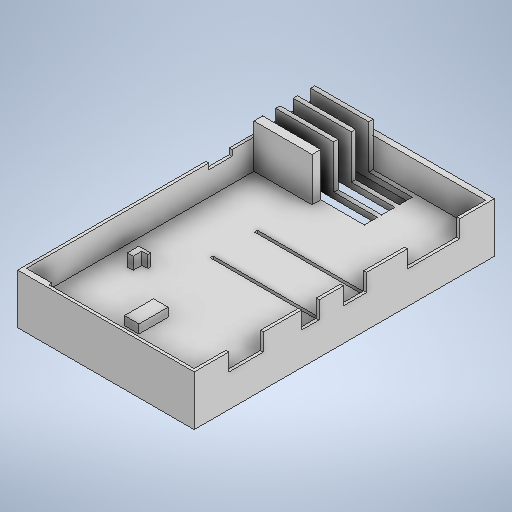
# Autodesk Inventor part: middle plate
Saved by Autodesk Inventor 2025.2 (Build 292293000, 293)
## iProperties
Created: 2025-04-04
Part Number: middle plate
Material: Generic
Document SubType Name: Modeling
Designer: joaki
Density: 1 g/cm^3
Appearance: Default
Author: joaki
Autodesk Inventor part; units mm, degrees
ref_plane "YZ Plane" through (0, 0, 0) normal (1, 0, 0) x (0, 1, 0)
ref_plane "XZ Plane" through (0, 0, 0) normal (0, 1, 0) x (-1, 0, 0)
ref_plane "XY Plane" through (0, 0, 0) normal (0, 0, 1) x (1, 0, 0)
sketch "Sketch1" plane through (0, 0, 0) normal (0, 1, 0) x (-1, 0, 0)
  line L0 (52.472, 79.0905) -> (-20.2681, 79.0905)
  line L1 (-20.2681, 79.0905) -> (-20.2681, -75.7549)
  line L2 (-20.2681, -75.7549) -> (52.472, -75.7549)
  line L3 (52.472, -75.7549) -> (52.472, 79.0905)
  line L4 (21.2319, -3.7723) -> (-15.2681, -3.7723)
  line L5 (-15.2681, -3.7723) -> (-15.2681, -4.7723)
  line L6 (-15.2681, -4.7723) -> (21.2319, -4.7723)
  line L7 (21.2319, -4.7723) -> (21.2319, -3.7723)
  line L8 (21.2319, -19.0703) -> (-15.2681, -19.0703)
  line L9 (-15.2681, -19.0703) -> (-15.2681, -20.0703)
  line L10 (-15.2681, -20.0703) -> (21.2319, -20.0703)
  line L11 (21.2319, -20.0703) -> (21.2319, -19.0703)
  point P0 (0, 0)
  point P1 (-15.2681, -4.2723)
  dimension "d0" = 36.5
  dimension "d1" = 1
  dimension "d2" = 1
  dimension "d3" = 36.5
  dimension "d4" = 14.298
  dimension "d7" = 5
  constraints: 24 end point, 6 parallel, 3 horizontal, 3 perpendicular, 1 midpoint
  measures "d0" distance of L5.end L6.end
  measures "d1" distance of L6.end L4.start
  measures "d2" distance of L10.end L8.start
  measures "d3" distance of L9.end L10.end
  measures "d4" distance between parallel lines of L6 L8
  measures "d7" distance from line of point (-15.268, -4.272) L1
extrude "Extrusion1" add sketch "Sketch1" along normal blind 2
sketch "Sketch3" plane through (0, 2, 0) normal (0, 1, 0) x (1, 0, 0)
  line L0 (20.2681, -79.0905) -> (20.2681, 75.7549) projected
  line L1 (20.2681, -79.0905) -> (19.2681, -79.0905)
  line L2 (19.2681, -79.0905) -> (19.2681, 75.7549)
  line L3 (19.2681, 75.7549) -> (20.2681, 75.7549)
  line L4 (20.2681, 75.7549) -> (20.2681, -79.0905)
  line L5 (20.2681, 75.7549) -> (-52.472, 75.7549) projected
  line L6 (-52.472, -79.0905) -> (20.2681, -79.0905) projected
  point P0 (0, 0)
  point P1 (19.7681, 75.7549)
  point P2 (19.7681, -79.0905)
  dimension "d8" = 1
  dimension "d9" = 0
  dimension "d10" = 0
  constraints: 8 end point, 2 midpoint, 2 parallel, 1 horizontal, 1 perpendicular, 1 point on line
  measures "d8" distance between parallel lines of L2 L0
  measures "d9" distance from line of L5 point (19.768, 75.755)
  measures "d10" distance from line of L6 point (19.768, -79.09)
extrude "Extrusion2" add sketch "Sketch3" along normal blind 4.2
sketch "Sketch5" plane through (0, 2, 0) normal (0, 1, 0) x (1, 0, 0)
  line L0 (19.2681, -79.0905) -> (19.2681, 75.7549) projected
  line L1 (17.2681, -9.2277) -> (19.2681, -9.2277)
  line L2 (19.2681, -9.2277) -> (19.2681, -11.2277)
  line L3 (19.2681, -11.2277) -> (17.2681, -11.2277)
  line L4 (17.2681, -11.2277) -> (17.2681, -9.2277)
  line L5 (15.2681, 3.7723) -> (-21.2319, 3.7723) projected
  line L6 (17.2681, -43.2277) -> (19.2681, -43.2277)
  line L7 (19.2681, -43.2277) -> (19.2681, -41.2277)
  line L8 (19.2681, -41.2277) -> (17.2681, -41.2277)
  line L9 (17.2681, -41.2277) -> (17.2681, -43.2277)
  line L10 (-32.7319, -9.2277) -> (-30.7319, -9.2277)
  line L11 (-30.7319, -9.2277) -> (-30.7319, -13.2277)
  line L12 (-30.7319, -13.2277) -> (-32.7319, -13.2277)
  line L13 (-32.7319, -13.2277) -> (-32.7319, -9.2277)
  line L14 (-30.7319, -9.2277) -> (-28.7319, -9.2277)
  line L15 (-28.7319, -9.2277) -> (-28.7319, -11.2277)
  line L16 (-28.7319, -11.2277) -> (-30.7319, -11.2277)
  line L17 (-30.7319, -11.2277) -> (-30.7319, -9.2277)
  line L18 (18.2681, -41.2277) -> (18.2681, -11.2277)
  line L19 (18.2681, -26.2277) -> (-4.7702, -26.2277)
  line L20 (-32.7319, -43.2277) -> (-30.7319, -43.2277)
  line L21 (-30.7319, -43.2277) -> (-30.7319, -39.2277)
  line L22 (-30.7319, -39.2277) -> (-32.7319, -39.2277)
  line L23 (-32.7319, -39.2277) -> (-32.7319, -43.2277)
  line L24 (-30.7319, -43.2277) -> (-28.7319, -43.2277)
  line L25 (-28.7319, -43.2277) -> (-28.7319, -41.2277)
  line L26 (-28.7319, -41.2277) -> (-30.7319, -41.2277)
  line L27 (-30.7319, -41.2277) -> (-30.7319, -43.2277)
  line L28 (-28.7319, -41.2277) -> (17.2681, -41.2277)
  line L29 (17.2681, -41.2277) -> (17.2681, -43.2277)
  line L30 (17.2681, -43.2277) -> (-28.7319, -43.2277)
  line L31 (-28.7319, -43.2277) -> (-28.7319, -41.2277)
  point P0 (0, 0)
  point P1 (18.2681, -9.2277)
  point P2 (18.2681, -43.2277)
  point P3 (19.2681, -42.2277)
  point P4 (17.2681, -42.2277)
  point P5 (-31.7319, -9.2277)
  point P6 (-31.7319, -13.2277)
  point P7 (17.2681, -10.2277)
  point P8 (-31.7319, -43.2277)
  point P9 (-31.7319, -39.2277)
  dimension "d57" = 12
  dimension "d13" = 2
  dimension "d14" = 2
  dimension "d15" = 13
  dimension "d18" = 2
  dimension "d19" = 2
  dimension "d20" = 0
  dimension "d21" = 30
  dimension "d22" = 2
  dimension "d23" = 4
  dimension "d24" = 48
  dimension "d25" = 0
  dimension "d26" = 2
  constraints: 60 end point, 10 midpoint, 10 parallel, 9 symmetric about line, 6 horizontal, 5 perpendicular, 1 point on line
  measures "d13" distance of L1.start L1.end
  measures "d14" distance of L3.end L1.start
  measures "d15" distance from line of point (18.268, -9.228) L5
  measures "d18" distance of point (18.268, -43.228) L18.start
  measures "d19" distance of point (19.268, -42.228) point (17.268, -42.228)
  measures "d20" distance from line of L0 point (19.268, -42.228)
  measures "d21" distance of L18.end L18.start
  measures "d22" distance of L11.end L12.end
  measures "d23" distance of point (-31.732, -9.228) point (-31.732, -13.228)
  measures "d24" distance from line of point (17.268, -10.228) L11
  measures "d25" distance between parallel lines of L1 L10
  measures "d26" distance of L15.end L16.end
extrude "Extrusion3" add sketch "Sketch5" along normal blind 4.2 contours L6 L9 L8 L0 | L30 L25 L28 L9 | L3 L4 L1 L0 | L24 L21 L26 L25 | L20 L23 L22 L21 | L10 L11 L12 L13 | L14 L15 L16 L11
sketch "Sketch6" plane through (0, 2, 0) normal (0, 1, 0) x (1, 0, 0)
  line L0 (19.2681, -11.2277) -> (17.2681, -11.2277) projected
  line L1 (17.2681, -11.2277) -> (17.2681, -41.2277)
  line L2 (17.2681, -26.2277) -> (-23.5137, -26.2277)
  line L3 (-15.7319, -21.2277) -> (-10.7319, -21.2277)
  line L4 (-10.7319, -21.2277) -> (-10.7319, -31.2277)
  line L5 (-10.7319, -31.2277) -> (-15.7319, -31.2277)
  line L6 (-15.7319, -31.2277) -> (-15.7319, -21.2277)
  line L7 (-30.7319, -13.2277) -> (-30.7319, -11.2277) projected
  point P0 (0, 0)
  point P1 (-30.7319, -12.2277)
  dimension "d27" = 5
  dimension "d28" = 5
  dimension "d29" = 15
  dimension "d30" = 5
  constraints: 12 end point, 2 horizontal, 2 midpoint, 2 parallel, 1 perpendicular
  measures "d27" distance between parallel lines of L2 L5
  measures "d28" distance between parallel lines of L2 L3
  measures "d29" distance from line of point (-30.732, -12.228) L6
  measures "d30" distance between parallel lines of L4 L6
extrude "Extrusion4" add sketch "Sketch6" along normal blind 3
sketch "Sketch7" plane through (0, 6.2, 0) normal (0, 1, 0) x (1, 0, 0)
  line L0 (17.2681, -41.2277) -> (17.2681, -43.2277) projected
  line L1 (17.2681, -43.2277) -> (20.4293, -43.2277)
  line L2 (20.4293, -43.2277) -> (20.4293, -79.0905)
  line L3 (20.4293, -79.0905) -> (17.2681, -79.0905)
  line L4 (17.2681, -79.0905) -> (17.2681, -43.2277)
  line L5 (20.4293, -43.2277) -> (-77.3066, -43.2277)
  line L6 (-77.3066, -43.2277) -> (-77.3066, -92.2716)
  line L7 (-77.3066, -92.2716) -> (20.4293, -92.2716)
  line L8 (20.4293, -92.2716) -> (20.4293, -43.2277)
  point P0 (0, 0)
  constraints: 16 end point, 4 parallel, 2 horizontal, 2 perpendicular
extrude "Extrusion5" cut sketch "Sketch7" against normal through all
sketch "Sketch8" plane through (0, 6.2, 0) normal (0, 1, 0) x (1, 0, 0)
  line L0 (19.2681, -9.2277) -> (19.2681, 75.7549) projected
  line L1 (20.2681, -43.2277) -> (20.2681, 75.7549) projected
  line L2 (19.2681, -6.2277) -> (20.2681, -6.2277)
  line L3 (20.2681, -6.2277) -> (20.2681, -0.2277)
  line L4 (20.2681, -0.2277) -> (19.2681, -0.2277)
  line L5 (19.2681, -0.2277) -> (19.2681, -6.2277)
  line L6 (19.2681, -9.2277) -> (17.2681, -9.2277) projected
  line L7 (19.2681, -0.2277) -> (20.2681, -0.2277)
  line L8 (20.2681, -0.2277) -> (20.2681, 8.1723)
  line L9 (20.2681, 8.1723) -> (19.2681, 8.1723)
  line L10 (19.2681, 8.1723) -> (19.2681, -0.2277)
  line L11 (19.2681, -6.2277) -> (20.2681, -6.2277)
  line L12 (20.2681, -6.2277) -> (20.2681, -11.9269)
  line L13 (20.2681, -11.9269) -> (19.2681, -11.9269)
  line L14 (19.2681, -11.9269) -> (19.2681, -6.2277)
  line L15 (19.2681, -9.2277) -> (20.2681, -9.2277)
  line L16 (20.2681, -9.2277) -> (20.2681, -19.4277)
  line L17 (20.2681, -19.4277) -> (19.2681, -19.4277)
  line L18 (19.2681, -19.4277) -> (19.2681, -9.2277)
  line L19 (19.2681, 8.1723) -> (20.2681, 8.1723)
  line L20 (20.2681, 8.1723) -> (20.2681, 15.1723)
  line L21 (20.2681, 15.1723) -> (19.2681, 15.1723)
  line L22 (19.2681, 15.1723) -> (19.2681, 8.1723)
  line L23 (19.2681, 15.1723) -> (20.2681, 15.1723)
  line L24 (20.2681, 15.1723) -> (20.2681, 30.1723)
  line L25 (20.2681, 30.1723) -> (19.2681, 30.1723)
  line L26 (19.2681, 30.1723) -> (19.2681, 15.1723)
  line L27 (19.2681, -19.4277) -> (20.2681, -19.4277)
  line L28 (20.2681, -19.4277) -> (20.2681, -31.3277)
  line L29 (20.2681, -31.3277) -> (19.2681, -31.3277)
  line L30 (19.2681, -31.3277) -> (19.2681, -19.4277)
  line L31 (19.2681, -31.3277) -> (20.2681, -31.3277)
  line L32 (20.2681, -31.3277) -> (20.2681, -43.2277)
  line L33 (20.2681, -43.2277) -> (19.2681, -43.2277)
  line L34 (19.2681, -43.2277) -> (19.2681, -31.3277)
  line L35 (19.2681, 30.1723) -> (20.2681, 30.1723)
  line L36 (20.2681, 30.1723) -> (20.2681, 45.1723)
  line L37 (20.2681, 45.1723) -> (19.2681, 45.1723)
  line L38 (19.2681, 45.1723) -> (19.2681, 30.1723)
  line L39 (19.2681, 45.1723) -> (20.2681, 45.1723)
  line L40 (20.2681, 45.1723) -> (20.2681, 55.138)
  line L41 (20.2681, 55.138) -> (19.2681, 55.138)
  line L42 (19.2681, 55.138) -> (19.2681, 45.1723)
  line L43 (19.2681, 55.138) -> (20.2681, 55.138)
  line L44 (20.2681, 55.138) -> (20.2681, 75.7549)
  line L45 (20.2681, 75.7549) -> (19.2681, 75.7549)
  line L46 (19.2681, 75.7549) -> (19.2681, 55.138)
  line L47 (-52.472, 75.7549) -> (-52.472, -43.2277) projected
  line L48 (19.2681, 75.7549) -> (-52.472, 75.7549)
  line L49 (-52.472, 75.7549) -> (-52.472, 73.7549)
  line L50 (-52.472, 73.7549) -> (19.2681, 73.7549)
  line L51 (19.2681, 73.7549) -> (19.2681, 75.7549)
  line L52 (-52.472, -43.2277) -> (-32.7319, -43.2277) projected
  line L53 (-52.472, 73.7549) -> (-51.472, 73.7549)
  line L54 (-51.472, 73.7549) -> (-51.472, -43.2277)
  line L55 (-51.472, -43.2277) -> (-52.472, -43.2277)
  line L56 (-52.472, -43.2277) -> (-52.472, 73.7549)
  line L57 (19.2681, -41.2277) -> (-30.7319, -41.2277) projected
  line L58 (-51.472, -43.2277) -> (19.2681, -43.2277)
  line L59 (19.2681, -43.2277) -> (19.2681, -41.2277)
  line L60 (19.2681, -41.2277) -> (-51.472, -41.2277)
  line L61 (-51.472, -41.2277) -> (-51.472, -43.2277)
  point P0 (0, 0)
  point P1 (19.7681, -0.2277)
  point P2 (19.7681, -6.2277)
  point P3 (18.2681, -9.2277)
  point P4 (19.7681, 8.1723)
  point P5 (19.7681, -0.2277)
  point P6 (19.7681, -9.2277)
  point P7 (19.7681, -19.4277)
  point P8 (19.7681, 15.1723)
  point P9 (19.7681, 8.1723)
  point P10 (19.2681, 30.1723)
  point P11 (19.7681, -19.4277)
  point P12 (19.7681, -31.3277)
  point P13 (19.7681, 30.1723)
  point P14 (19.7681, 15.1723)
  point P15 (19.7681, 45.1723)
  point P16 (19.7681, 30.1723)
  dimension "d35" = 6
  dimension "d36" = 3
  dimension "d39" = 8.4
  dimension "d40" = 10.2
  dimension "d41" = 7
  dimension "d42" = 11.9
  dimension "d79" = 15
  dimension "d80" = 15
  dimension "d87" = 2
  dimension "d88" = 1
  constraints: 112 end point, 28 parallel, 15 midpoint, 14 horizontal, 14 perpendicular, 3 point on line, 10 other
  measures "d35" distance of point (19.768, -0.228) point (19.768, -6.228)
  measures "d36" vertical distance of point (18.268, -9.228) point (19.768, -6.228)
  measures "d39" distance of point (19.768, 8.172) point (19.768, -0.228)
  measures "d40" distance of point (19.768, -9.228) point (19.768, -19.428)
  measures "d41" distance of point (19.768, 15.172) point (19.768, 8.172)
  measures "d42" distance of point (19.768, -19.428) point (19.768, -31.328)
  measures "d79" distance of point (19.768, 30.172) point (19.768, 15.172)
  measures "d80" distance of point (19.768, 45.172) point (19.768, 30.172)
  measures "d87" distance between parallel lines of L48 L50
  measures "d88" distance between parallel lines of L56 L54
extrude "Extrusion6" add sketch "Sketch8" along normal blind 6 contours L15 L1 L13 L14 | L0 L2 L1 L15 | L13 L1 L17 L18 | L0 L9 L1 L4 | L29 L1 L33 L34 | L0 L25 L1 L21 | L0 L41 L1 L37
sketch "Sketch9" plane through (0, 0, 0) normal (0, -1, 0) x (1, 0, 0)
  line L0 (-10.4819, -25.0703) -> (4.5181, -25.0703)
  line L1 (4.5181, -25.0703) -> (4.5181, -26.0703)
  line L2 (4.5181, -26.0703) -> (-10.4819, -26.0703)
  line L3 (-10.4819, -26.0703) -> (-10.4819, -25.0703)
  line L4 (-21.2319, -20.0703) -> (15.2681, -20.0703) projected
  line L5 (-2.9819, -20.0703) -> (-2.9819, -60.9317)
  line L6 (-10.4819, -29.1703) -> (4.5181, -29.1703)
  line L7 (4.5181, -29.1703) -> (4.5181, -28.1703)
  line L8 (4.5181, -28.1703) -> (-10.4819, -28.1703)
  line L9 (-10.4819, -28.1703) -> (-10.4819, -29.1703)
  line L10 (-10.4819, -32.2703) -> (4.5181, -32.2703)
  line L11 (4.5181, -32.2703) -> (4.5181, -31.2703)
  line L12 (4.5181, -31.2703) -> (-10.4819, -31.2703)
  line L13 (-10.4819, -31.2703) -> (-10.4819, -32.2703)
  line L14 (-10.4819, -35.3703) -> (4.5181, -35.3703)
  line L15 (4.5181, -35.3703) -> (4.5181, -34.3703)
  line L16 (4.5181, -34.3703) -> (-10.4819, -34.3703)
  line L17 (-10.4819, -34.3703) -> (-10.4819, -35.3703)
  line L18 (-10.4819, -38.4703) -> (4.5181, -38.4703)
  line L19 (4.5181, -38.4703) -> (4.5181, -37.4703)
  line L20 (4.5181, -37.4703) -> (-10.4819, -37.4703)
  line L21 (-10.4819, -37.4703) -> (-10.4819, -38.4703)
  point P0 (0, 0)
  point P1 (-10.4819, -25.5703)
  point P2 (4.5181, -25.5703)
  dimension "d43" = 1
  dimension "d44" = 15
  dimension "d45" = 7.5
  dimension "d46" = 5
  dimension "d47" = 1
  dimension "d48" = 1
  dimension "d49" = 1
  dimension "d50" = 1
  dimension "d51" = 2.1
  dimension "d52" = 2.1
  dimension "d53" = 2.1
  dimension "d54" = 2.1
  constraints: 42 end point, 10 parallel, 6 point on line, 5 horizontal, 5 perpendicular, 3 midpoint, 1 vertical
  measures "d43" distance between parallel lines of L0 L2
  measures "d44" distance of point (-10.482, -25.57) point (4.518, -25.57)
  measures "d45" distance from line of L5 point (-10.482, -25.57)
  measures "d46" distance between parallel lines of L4 L0
  measures "d47" distance between parallel lines of L8 L6
  measures "d48" distance between parallel lines of L12 L10
  measures "d49" distance between parallel lines of L16 L14
  measures "d50" distance between parallel lines of L20 L18
  measures "d51" distance between parallel lines of L2 L8
  measures "d52" distance between parallel lines of L6 L12
  measures "d53" distance between parallel lines of L10 L16
  measures "d54" distance between parallel lines of L14 L20
extrude "Extrusion7" add sketch "Sketch9" along normal blind 2.1
sketch "Sketch10" plane through (0, 2, 0) normal (0, 1, 0) x (1, 0, 0)
  line L0 (-52.472, 75.7549) -> (-52.472, -43.2277) projected
  line L1 (19.2681, 75.7549) -> (-52.472, 75.7549) projected
  line L2 (-52.472, -43.2277) -> (-40.472, -43.2277)
  line L3 (-40.472, -43.2277) -> (-40.472, 75.7549)
  line L4 (-40.472, 75.7549) -> (-52.472, 75.7549)
  line L5 (-52.472, 75.7549) -> (-52.472, -43.2277)
  point P0 (0, 0)
  dimension "d57" = 12
  constraints: 8 end point, 2 parallel, 1 horizontal, 1 perpendicular, 1 point on line
  measures "d57" distance between parallel lines of L0 L3
extrude "Extrusion8" cut sketch "Sketch10" against normal blind 2.1
sketch "Sketch11" plane through (0, 2, 0) normal (0, 1, 0) x (1, 0, 0)
  line L0 (-32.7319, -43.2277) -> (-32.7319, -39.2277) projected
  line L1 (-40.472, -43.2277) -> (-40.472, 75.7549) projected
  line L2 (-32.7319, -43.2277) -> (-40.472, -43.2277)
  line L3 (-40.472, -43.2277) -> (-40.472, -41.2277)
  line L4 (-40.472, -41.2277) -> (-32.7319, -41.2277)
  line L5 (-32.7319, -41.2277) -> (-32.7319, -43.2277)
  line L6 (19.2681, 75.7549) -> (-40.472, 75.7549) projected
  line L7 (-40.472, -41.2277) -> (-39.472, -41.2277)
  line L8 (-39.472, -41.2277) -> (-39.472, 75.7549)
  line L9 (-39.472, 75.7549) -> (-40.472, 75.7549)
  line L10 (-40.472, 75.7549) -> (-40.472, -41.2277)
  point P0 (0, 0)
  dimension "d60" = 2
  dimension "d61" = 1
  constraints: 16 end point, 4 parallel, 2 horizontal, 2 perpendicular, 2 point on line
  measures "d60" distance between parallel lines of L4 L2
  measures "d61" distance between parallel lines of L1 L8
extrude "Extrusion9" add sketch "Sketch11" along normal blind 4.2
sketch "Sketch12" plane through (0, 2, 0) normal (0, 1, 0) x (1, 0, 0)
  line L0 (-39.472, 75.7549) -> (-39.472, -41.2277) projected
  line L1 (-39.472, 37.0703) -> (-19.472, 37.0703)
  line L2 (-19.472, 37.0703) -> (-19.472, 40.0703)
  line L3 (-19.472, 40.0703) -> (-39.472, 40.0703)
  line L4 (-39.472, 40.0703) -> (-39.472, 37.0703)
  line L5 (-21.2319, 20.0703) -> (15.2681, 20.0703) projected
  line L6 (-19.472, 43.0703) -> (-39.472, 43.0703)
  line L7 (-39.472, 43.0703) -> (-39.472, 46.0703)
  line L8 (-39.472, 46.0703) -> (-19.472, 46.0703)
  line L9 (-19.472, 46.0703) -> (-19.472, 43.0703)
  line L10 (-19.472, 49.0703) -> (-39.472, 49.0703)
  line L11 (-39.472, 49.0703) -> (-39.472, 52.0703)
  line L12 (-39.472, 52.0703) -> (-19.472, 52.0703)
  line L13 (-19.472, 52.0703) -> (-19.472, 49.0703)
  line L14 (-19.472, 55.0703) -> (-39.472, 55.0703)
  line L15 (-39.472, 55.0703) -> (-39.472, 58.0703)
  line L16 (-39.472, 58.0703) -> (-19.472, 58.0703)
  line L17 (-19.472, 58.0703) -> (-19.472, 55.0703)
  point P0 (0, 0)
  point P1 (-39.472, 38.5703)
  point P2 (-19.472, 38.5703)
  point P3 (-29.472, 37.0703)
  point P4 (-29.472, 46.0703)
  point P5 (-39.472, 43.0703)
  dimension "d64" = 3
  dimension "d65" = 20
  dimension "d66" = 17
  dimension "d67" = 3
  dimension "d68" = 3
  dimension "d69" = 3
  dimension "d70" = 3
  dimension "d71" = 3
  dimension "d72" = 3
  constraints: 32 end point, 8 parallel, 6 point on line, 4 horizontal, 4 midpoint, 4 perpendicular
  measures "d64" distance between parallel lines of L3 L1
  measures "d65" distance of point (-39.472, 38.57) point (-19.472, 38.57)
  measures "d66" distance from line of point (-29.472, 37.07) L5
  measures "d67" distance from line of point (-29.472, 46.07) L6
  measures "d68" distance between parallel lines of L12 L10
  measures "d69" distance between parallel lines of L16 L14
  measures "d70" distance between parallel lines of L6 L3
  measures "d71" distance between parallel lines of L10 L8
  measures "d72" distance between parallel lines of L14 L12
extrude "Extrusion10" add sketch "Sketch12" along normal blind 15
sketch "Sketch13" plane through (0, 2, 0) normal (0, 1, 0) x (1, 0, 0)
  line L0 (-39.472, 40.0703) -> (-39.472, 43.0703) projected
  line L1 (-39.472, 40.0703) -> (-4.472, 40.0703)
  line L2 (-4.472, 40.0703) -> (-4.472, 43.0703)
  line L3 (-4.472, 43.0703) -> (-39.472, 43.0703)
  line L4 (-39.472, 43.0703) -> (-39.472, 40.0703)
  line L5 (-19.472, 46.0703) -> (-39.472, 46.0703) projected
  line L6 (-39.472, 46.0703) -> (-4.472, 46.0703)
  line L7 (-4.472, 46.0703) -> (-4.472, 49.0703)
  line L8 (-4.472, 49.0703) -> (-39.472, 49.0703)
  line L9 (-39.472, 49.0703) -> (-39.472, 46.0703)
  line L10 (-19.472, 52.0703) -> (-39.472, 52.0703) projected
  line L11 (-39.472, 52.0703) -> (-4.472, 52.0703)
  line L12 (-4.472, 52.0703) -> (-4.472, 55.0703)
  line L13 (-4.472, 55.0703) -> (-39.472, 55.0703)
  line L14 (-39.472, 55.0703) -> (-39.472, 52.0703)
  line L15 (-39.472, 46.0703) -> (-39.472, 49.0703) projected
  line L16 (-39.472, 55.0703) -> (-19.472, 55.0703) projected
  point P0 (0, 0)
  point P1 (-39.472, 41.5703)
  point P2 (-4.472, 41.5703)
  point P3 (-39.472, 47.5703)
  point P4 (-4.472, 47.5703)
  dimension "d75" = 35
  dimension "d76" = 35
  dimension "d81" = 0
  constraints: 24 end point, 6 parallel, 4 midpoint, 3 horizontal, 3 perpendicular, 1 point on line
  measures "d75" distance of point (-39.472, 41.57) point (-4.472, 41.57)
  measures "d76" distance of point (-39.472, 47.57) point (-4.472, 47.57)
  measures "d81" distance between parallel lines of L16 L13
extrude "Extrusion11" cut sketch "Sketch13" against normal blind 12
sketch "Sketch14" plane through (0, 2, 0) normal (0, 1, 0) x (1, 0, 0)
  line L0 (-19.472, 58.0703) -> (-39.472, 58.0703) projected
  line L1 (19.2681, -9.2277) -> (19.2681, 75.7549) projected
  line L2 (-39.472, 58.0703) -> (19.2681, 58.0703)
  line L3 (19.2681, 58.0703) -> (19.2681, 60.0703)
  line L4 (19.2681, 60.0703) -> (-39.472, 60.0703)
  line L5 (-39.472, 60.0703) -> (-39.472, 58.0703)
  point P0 (0, 0)
  point P1 (19.2681, 58.0703)
  dimension "d82" = 2
  constraints: 8 end point, 2 parallel, 1 horizontal, 1 perpendicular, 1 point on line
  measures "d82" distance between parallel lines of L4 L2
extrude "Extrusion12" add sketch "Sketch14" along normal blind 4.2
sketch "Sketch15" plane through (0, 6.2, 0) normal (0, 1, 0) x (1, 0, 0)
  line L0 (-40.472, 75.7549) -> (-40.472, -43.2277) projected
  line L1 (-40.472, 75.7549) -> (24.3704, 75.7549)
  line L2 (24.3704, 75.7549) -> (24.3704, 60.0703)
  line L3 (24.3704, 60.0703) -> (-40.472, 60.0703)
  line L4 (-40.472, 60.0703) -> (-40.472, 75.7549)
  point P0 (0, 0)
  constraints: 8 end point, 2 parallel, 1 horizontal, 1 perpendicular
extrude "Extrusion13" cut sketch "Sketch15" against normal through all
sketch "Sketch16" plane through (0, 6.2, 0) normal (0, 1, 0) x (1, 0, 0)
  line L0 (19.2681, 55.138) -> (19.2681, 45.1723) projected
  line L1 (20.2681, 60.0703) -> (-40.472, 60.0703) projected
  line L2 (19.2681, 55.138) -> (20.2681, 55.138)
  line L3 (20.2681, 55.138) -> (20.2681, 60.0703)
  line L4 (20.2681, 60.0703) -> (19.2681, 60.0703)
  line L5 (19.2681, 60.0703) -> (19.2681, 55.138)
  line L6 (-39.472, 55.0703) -> (-39.472, 58.0703) projected
  line L7 (19.2681, 60.0703) -> (-39.472, 60.0703)
  line L8 (-39.472, 60.0703) -> (-39.472, 58.0703)
  line L9 (-39.472, 58.0703) -> (19.2681, 58.0703)
  line L10 (19.2681, 58.0703) -> (19.2681, 60.0703)
  line L11 (-40.472, 60.0703) -> (-40.472, -43.2277) projected
  line L12 (-40.472, 60.0703) -> (-39.472, 60.0703)
  line L13 (-39.472, 60.0703) -> (-39.472, -43.2277)
  line L14 (-39.472, -43.2277) -> (-40.472, -43.2277)
  line L15 (-40.472, -43.2277) -> (-40.472, 60.0703)
  line L16 (-32.7319, -41.2277) -> (-39.472, -41.2277) projected
  line L17 (-39.472, -41.2277) -> (19.2681, -41.2277)
  line L18 (19.2681, -41.2277) -> (19.2681, -43.2277)
  line L19 (19.2681, -43.2277) -> (-39.472, -43.2277)
  line L20 (-39.472, -43.2277) -> (-39.472, -41.2277)
  point P0 (0, 0)
  constraints: 32 end point, 8 parallel, 4 horizontal, 4 perpendicular, 3 point on line
extrude "Extrusion14" add sketch "Sketch16" along normal blind 6
sketch "Sketch17" plane through (0, 0, 0) normal (0, -1, 0) x (1, 0, 0)
  line L0 (-40.472, 43.2277) -> (20.2681, 43.2277) projected
  line L1 (20.2681, -60.0703) -> (-40.472, -60.0703) projected
  line L2 (20.2681, 43.2277) -> (19.2681, 43.2277)
  line L3 (19.2681, 43.2277) -> (19.2681, -60.0703)
  line L4 (19.2681, -60.0703) -> (20.2681, -60.0703)
  line L5 (20.2681, -60.0703) -> (20.2681, 43.2277)
  line L6 (-40.472, -60.0703) -> (-40.472, 43.2277) projected
  line L7 (19.2681, -60.0703) -> (-40.472, -60.0703)
  line L8 (-40.472, -60.0703) -> (-40.472, -58.0703)
  line L9 (-40.472, -58.0703) -> (19.2681, -58.0703)
  line L10 (19.2681, -58.0703) -> (19.2681, -60.0703)
  line L11 (19.2681, 43.2277) -> (-40.472, 43.2277)
  line L12 (-40.472, 43.2277) -> (-40.472, 41.2277)
  line L13 (-40.472, 41.2277) -> (19.2681, 41.2277)
  line L14 (19.2681, 41.2277) -> (19.2681, 43.2277)
  point P0 (0, 0)
  point P1 (19.2681, -58.0703)
  dimension "d91" = 1
  dimension "d92" = 2
  dimension "d93" = 2
  constraints: 24 end point, 6 parallel, 3 horizontal, 3 perpendicular, 3 point on line
  measures "d91" distance between parallel lines of L5 L3
  measures "d92" distance between parallel lines of L1 L9
  measures "d93" distance between parallel lines of L0 L13
extrude "Extrusion15" add sketch "Sketch17" along normal blind 5 contours L0 L3 L13 L6 | L0 L5 L1 L3 | L9 L3 L1 L6
sketch "Sketch18" plane through (0, 0, 0) normal (0, -1, 0) x (1, 0, 0)
  line L0 (-30.7319, 41.2277) -> (19.2681, 41.2277) projected
  line L1 (19.2681, 41.2277) -> (4.79, 41.2277)
  line L2 (4.79, 41.2277) -> (4.79, 5.2277)
  line L3 (4.79, 5.2277) -> (19.2681, 5.2277)
  line L4 (19.2681, 5.2277) -> (19.2681, 41.2277)
  line L5 (-40.472, 41.2277) -> (-40.472, -58.0703) projected
  line L6 (19.2681, 5.2277) -> (-40.472, 5.2277)
  line L7 (-40.472, 5.2277) -> (-40.472, 4.2277)
  line L8 (-40.472, 4.2277) -> (19.2681, 4.2277)
  line L9 (19.2681, 4.2277) -> (19.2681, 5.2277)
  point P0 (0, 0)
  point P1 (12.0291, 5.2277)
  point P2 (12.0291, 41.2277)
  point P3 (4.79, 5.2277)
  dimension "d96" = 36
  dimension "d97" = 1
  constraints: 16 end point, 4 parallel, 2 horizontal, 2 midpoint, 2 perpendicular, 1 point on line
  measures "d96" distance of point (12.029, 5.228) point (12.029, 41.228)
  measures "d97" distance between parallel lines of L8 L6
extrude "Extrusion16" add sketch "Sketch18" along normal blind 5 contours L3 L9 L8 L5 L6
sketch "Sketch19" plane through (0, 0, 0) normal (0, -1, 0) x (1, 0, 0)
  line L0 (-40.472, -60.0703) -> (-40.472, 43.2277) projected
  line L1 (-40.472, 4.2277) -> (-18.472, 4.2277)
  line L2 (-18.472, 4.2277) -> (-18.472, -17.7723)
  line L3 (-18.472, -17.7723) -> (-40.472, -17.7723)
  line L4 (-40.472, -17.7723) -> (-40.472, 4.2277)
  line L5 (-40.472, 4.2277) -> (19.2681, 4.2277) projected
  line L6 (-18.472, 4.2277) -> (-40.472, 4.2277)
  line L7 (-40.472, 4.2277) -> (-40.472, 2.2277)
  line L8 (-40.472, 2.2277) -> (-18.472, 2.2277)
  line L9 (-18.472, 2.2277) -> (-18.472, 4.2277)
  line L10 (-18.472, -17.7723) -> (-40.472, -17.7723)
  line L11 (-40.472, -17.7723) -> (-40.472, -15.7723)
  line L12 (-40.472, -15.7723) -> (-18.472, -15.7723)
  line L13 (-18.472, -15.7723) -> (-18.472, -17.7723)
  line L14 (-40.472, 2.2277) -> (-38.472, 2.2277)
  line L15 (-38.472, 2.2277) -> (-38.472, -1.9723)
  line L16 (-38.472, -1.9723) -> (-40.472, -1.9723)
  line L17 (-40.472, -1.9723) -> (-40.472, 2.2277)
  line L18 (-40.472, -15.7723) -> (-38.472, -15.7723)
  line L19 (-38.472, -15.7723) -> (-38.472, -11.5723)
  line L20 (-38.472, -11.5723) -> (-40.472, -11.5723)
  line L21 (-40.472, -11.5723) -> (-40.472, -15.7723)
  point P0 (0, 0)
  point P1 (-29.472, 4.2277)
  point P2 (-39.472, -15.7723)
  point P3 (-39.472, -11.5723)
  point P4 (-40.472, 0.1277)
  point P5 (-38.472, 0.1277)
  dimension "d100" = 0
  dimension "d101" = 22
  dimension "d102" = 22
  dimension "d103" = 2
  dimension "d104" = 2
  dimension "d107" = 2
  dimension "d108" = 4.2
  dimension "d109" = 4.2
  dimension "d110" = 2
  constraints: 40 end point, 10 parallel, 5 horizontal, 5 midpoint, 5 perpendicular, 3 point on line
  measures "d100" distance between parallel lines of L5 L1
  measures "d101" distance from line of point (-29.472, 4.228) L3
  measures "d102" distance between parallel lines of L0 L2
  measures "d103" distance between parallel lines of L3 L12
  measures "d104" distance between parallel lines of L6 L8
  measures "d107" distance between parallel lines of L4 L19
  measures "d108" distance of point (-39.472, -15.772) point (-39.472, -11.572)
  measures "d109" distance between parallel lines of L14 L16
  measures "d110" distance of point (-40.472, 0.128) point (-38.472, 0.128)
extrude "Extrusion17" add sketch "Sketch19" along normal blind 5.5 contours L0 L12 L2 L3 | L0 L20 L19 L12 | L0 L8 L15 L16 | L8 L0 L1 L2
sketch "Sketch20" plane through (0, 0, 0) normal (0, -1, 0) x (1, 0, 0)
  line L0 (-40.472, -60.0703) -> (-40.472, 43.2277) projected
  line L1 (-40.472, -58.0703) -> (19.2681, -58.0703) projected
  line L2 (-40.472, -17.7213) -> (-39.472, -17.7213)
  line L3 (-39.472, -17.7213) -> (-39.472, -58.0703)
  line L4 (-39.472, -58.0703) -> (-40.472, -58.0703)
  line L5 (-40.472, -58.0703) -> (-40.472, -17.7213)
  point P0 (0, 0)
  dimension "d111" = 1
  constraints: 8 end point, 2 parallel, 2 point on line, 1 horizontal, 1 perpendicular
  measures "d111" distance between parallel lines of L0 L3
extrude "Extrusion18" add sketch "Sketch20" along normal blind 5
sketch "Sketch21" plane through (0, 0, 0) normal (0, -1, 0) x (1, 0, 0)
  line L0 (-39.472, -40.0703) -> (-4.472, -40.0703) projected
  line L1 (-39.472, -40.0703) -> (-24.372, -40.0703)
  line L2 (-24.372, -40.0703) -> (-24.372, -39.0703)
  line L3 (-24.372, -39.0703) -> (-39.472, -39.0703)
  line L4 (-39.472, -39.0703) -> (-39.472, -40.0703)
  line L5 (-40.472, -17.7723) -> (-18.472, -17.7723) projected
  line L6 (-24.372, -39.0703) -> (-25.372, -39.0703)
  line L7 (-25.372, -39.0703) -> (-25.372, -17.7723)
  line L8 (-25.372, -17.7723) -> (-24.372, -17.7723)
  line L9 (-24.372, -17.7723) -> (-24.372, -39.0703)
  point P0 (0, 0)
  point P1 (-39.472, -39.5703)
  dimension "d114" = 15.1
  dimension "d115" = 1
  dimension "d116" = 1
  constraints: 16 end point, 4 parallel, 2 horizontal, 2 perpendicular, 1 midpoint, 1 point on line
  measures "d114" distance from line of point (-39.472, -39.57) L2
  measures "d115" distance between parallel lines of L0 L3
  measures "d116" distance between parallel lines of L9 L7
extrude "Extrusion19" add sketch "Sketch21" along normal blind 4
sketch "Sketch22" plane through (0, 0, 0) normal (0, -1, 0) x (1, 0, 0)
  line L0 (-25.372, -39.0703) -> (-39.472, -39.0703) projected
  line L1 (-39.472, -17.7723) -> (-39.472, -39.0703) projected
  line L2 (-25.372, -39.0703) -> (-39.472, -39.0703)
  line L3 (-39.472, -39.0703) -> (-39.472, -27.0703)
  line L4 (-39.472, -27.0703) -> (-25.372, -27.0703)
  line L5 (-25.372, -27.0703) -> (-25.372, -39.0703)
  point P0 (0, 0)
  point P1 (-32.422, -39.0703)
  point P2 (-32.422, -27.0703)
  dimension "d119" = 12
  constraints: 8 end point, 2 midpoint, 2 parallel, 1 horizontal, 1 perpendicular, 1 point on line
  measures "d119" distance of point (-32.422, -39.07) point (-32.422, -27.07)
extrude "Extrusion20" add sketch "Sketch22" along normal blind 2
sketch "Sketch25" plane through (0, 12.2, 0) normal (0, 1, 0) x (1, 0, 0)
  line L0 (-40.472, 17.7723) -> (-40.472, 60.0703) projected
  line L1 (-39.472, 39.0703) -> (-39.472, 27.0703) projected
  line L2 (-40.472, 21.5457) -> (-39.472, 21.5457)
  line L3 (-39.472, 21.5457) -> (-39.472, 29.5457)
  line L4 (-39.472, 29.5457) -> (-40.472, 29.5457)
  line L5 (-40.472, 29.5457) -> (-40.472, 21.5457)
  point P0 (0, 0)
  point P1 (-39.972, 29.5457)
  point P2 (-39.972, 21.5457)
  dimension "d124" = 8
  constraints: 8 end point, 2 midpoint, 2 parallel, 2 point on line, 1 horizontal, 1 perpendicular
  measures "d124" distance of point (-39.972, 29.546) point (-39.972, 21.546)
extrude "Extrusion21" cut sketch "Sketch25" against normal blind 2
sketch "Sketch26" plane through (0, 17, 0) normal (0, 1, 0) x (1, 0, 0)
  line L0 (-19.472, 55.0703) -> (-19.472, 58.0703) projected
  line L1 (-39.472, 55.0703) -> (-19.472, 55.0703)
  line L2 (-19.472, 55.0703) -> (-19.472, 56.5703)
  line L3 (-19.472, 56.5703) -> (-39.472, 56.5703)
  line L4 (-39.472, 56.5703) -> (-39.472, 55.0703)
  line L5 (-39.472, 46.0703) -> (-39.472, 49.0703) projected
  line L6 (-19.472, 49.0703) -> (-19.472, 52.0703) projected
  line L7 (-39.472, 49.0703) -> (-19.472, 49.0703)
  line L8 (-19.472, 49.0703) -> (-19.472, 50.5703)
  line L9 (-19.472, 50.5703) -> (-39.472, 50.5703)
  line L10 (-39.472, 50.5703) -> (-39.472, 49.0703)
  line L11 (-39.472, 43.0703) -> (-19.472, 43.0703) projected
  line L12 (-19.472, 43.0703) -> (-19.472, 46.0703) projected
  line L13 (-39.472, 43.0703) -> (-19.472, 43.0703)
  line L14 (-19.472, 43.0703) -> (-19.472, 44.5703)
  line L15 (-19.472, 44.5703) -> (-39.472, 44.5703)
  line L16 (-39.472, 44.5703) -> (-39.472, 43.0703)
  line L17 (-4.472, 55.0703) -> (-39.472, 55.0703) projected
  line L18 (-19.472, 56.5703) -> (-4.472, 56.5703)
  line L19 (-4.472, 56.5703) -> (-4.472, 55.0703)
  line L20 (-4.472, 55.0703) -> (-19.472, 55.0703)
  line L21 (-19.472, 55.0703) -> (-19.472, 56.5703)
  line L22 (-19.472, 50.5703) -> (-4.472, 50.5703)
  line L23 (-4.472, 50.5703) -> (-4.472, 49.0703)
  line L24 (-4.472, 49.0703) -> (-19.472, 49.0703)
  line L25 (-19.472, 49.0703) -> (-19.472, 50.5703)
  line L26 (-4.472, 43.0703) -> (-39.472, 43.0703) projected
  line L27 (-19.472, 44.5703) -> (-4.472, 44.5703)
  line L28 (-4.472, 44.5703) -> (-4.472, 43.0703)
  line L29 (-4.472, 43.0703) -> (-19.472, 43.0703)
  line L30 (-19.472, 43.0703) -> (-19.472, 44.5703)
  point P0 (0, 0)
  dimension "d127" = 1.5
  dimension "d128" = 1.5
  dimension "d129" = 1.5
  constraints: 48 end point, 12 parallel, 6 horizontal, 6 perpendicular, 3 midpoint, 1 point on line
  measures "d127" distance between parallel lines of L3 L1
  measures "d128" distance between parallel lines of L9 L7
  measures "d129" distance between parallel lines of L15 L11
extrude "Extrusion22" cut sketch "Sketch26" against normal through all
sketch "Sketch27" plane through (20.2681, 6.2, -45.1723) normal (1, 0, 0) x (0, 0, -1)
  line L0 (-30, 0) -> (-30, 6) projected
  line L1 (-30, 6) -> (-29, 6)
  line L2 (-29, 6) -> (-29, 0)
  line L3 (-29, 0) -> (-30, 0)
  line L4 (-30, 0) -> (-30, 6)
  point P0 (-45.1723, -6.2)
  dimension "d132" = 1
  constraints: 8 end point, 2 parallel, 1 horizontal, 1 perpendicular
  measures "d132" distance between parallel lines of L2 L0
extrude "Extrusion23" cut sketch "Sketch27" against normal blind 10
sketch "Sketch28" plane through (0, 6.2, 0) normal (0, 1, 0) x (1, 0, 0)
  line L0 (-30.7319, -11.2277) -> (-28.7319, -11.2277) projected
  line L1 (19.2681, -11.2277) -> (19.2681, -9.2277) projected
  line L2 (-30.7319, -11.2277) -> (19.2681, -11.2277)
  line L3 (19.2681, -11.2277) -> (19.2681, -10.2277)
  line L4 (19.2681, -10.2277) -> (-30.7319, -10.2277)
  line L5 (-30.7319, -10.2277) -> (-30.7319, -11.2277)
  point P0 (0, 0)
  constraints: 8 end point, 2 parallel, 1 horizontal, 1 midpoint, 1 perpendicular
extrude "Extrusion24" cut sketch "Sketch28" against normal blind 4.2
sketch "Sketch29" plane through (-25.372, -4, -17.7723) normal (-1, 0, 0) x (0, 0, 1)
  line L0 (-9.298, 4) -> (0, 4) projected
  line L1 (0, 0) -> (-21.298, 0) projected
  line L2 (0, 4) -> (-10.649, 4)
  line L3 (-10.649, 4) -> (-10.649, 0)
  line L4 (-10.649, 0) -> (0, 0)
  line L5 (0, 0) -> (0, 4)
  line L6 (-9.298, 2) -> (-21.298, 2) projected
  line L7 (-10.649, 0) -> (-21.298, 0)
  line L8 (-21.298, 0) -> (-21.298, 2)
  line L9 (-21.298, 2) -> (-10.649, 2)
  line L10 (-10.649, 2) -> (-10.649, 0)
  point P0 (17.7723, 4)
  point P1 (-10.649, 2)
  constraints: 16 end point, 4 parallel, 2 horizontal, 2 perpendicular, 1 midpoint
extrude "Extrusion25" cut sketch "Sketch29" against normal blind 4.2
sketch "Sketch30" plane through (0, 0, 0) normal (0, -1, 0) x (1, 0, 0)
  line L0 (-39.472, -27.0703) -> (-25.372, -27.0703) projected
  line L1 (-24.372, -28.4213) -> (-24.372, -39.0703) projected
  line L2 (-25.372, -27.0703) -> (-24.372, -27.0703)
  line L3 (-24.372, -27.0703) -> (-24.372, -28.4213)
  line L4 (-24.372, -28.4213) -> (-25.372, -28.4213)
  line L5 (-25.372, -28.4213) -> (-25.372, -27.0703)
  point P0 (0, 0)
  constraints: 8 end point, 2 parallel, 1 horizontal, 1 perpendicular
extrude "Extrusion26" add sketch "Sketch30" along normal blind 2
sketch "Sketch32" plane through (0, -5, 0) normal (0, -1, 0) x (1, 0, 0)
  line L0 (-40.472, 41.2277) -> (-40.472, 5.2277) projected
  line L1 (-40.472, 41.2277) -> (19.2681, 41.2277)
  line L2 (19.2681, 41.2277) -> (19.2681, 42.2277)
  line L3 (19.2681, 42.2277) -> (-40.472, 42.2277)
  line L4 (-40.472, 42.2277) -> (-40.472, 41.2277)
  point P0 (0, 0)
  dimension "d141" = 1
  constraints: 8 end point, 2 parallel, 1 horizontal, 1 perpendicular
  measures "d141" distance between parallel lines of L1 L3
extrude "Extrusion27" cut sketch "Sketch32" against normal blind 5
sketch "Sketch33" plane through (20.2681, 6.2, -8.1723) normal (1, 0, 0) x (0, 0, -1)
  line L0 (37, 6) -> (40, 6)
  line L1 (40, 6) -> (40, 0)
  line L2 (40, 0) -> (37, 0)
  line L3 (37, 0) -> (37, 6)
  point P0 (-8.1723, -6.2)
  dimension "d144" = 3
  constraints: 8 end point, 2 parallel, 1 horizontal, 1 perpendicular
  measures "d144" distance between parallel lines of L1 L3
extrude "Extrusion28" cut sketch "Sketch33" against normal blind 5
sketch "Sketch34" plane through (0, 12.2, 0) normal (0, 1, 0) x (1, 0, 0)
  line L0 (-30.7319, -41.2277) -> (-30.7319, -39.2277) projected
  line L1 (-40.472, -42.2277) -> (19.2681, -42.2277) projected
  line L2 (-30.7319, -41.2277) -> (19.2681, -41.2277)
  line L3 (19.2681, -41.2277) -> (19.2681, -42.2277)
  line L4 (19.2681, -42.2277) -> (-30.7319, -42.2277)
  line L5 (-30.7319, -42.2277) -> (-30.7319, -41.2277)
  point P0 (0, 0)
  point P1 (-30.7319, -42.2277)
  constraints: 8 end point, 2 parallel, 1 horizontal, 1 perpendicular
extrude "Extrusion29" cut sketch "Sketch34" against normal blind 10.2
body "Solid1"
